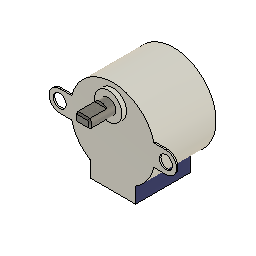
28BYJ-48 – 5V Stepper Motor (Autodesk Fusion 360 design; units mm, degrees)
Autodesk Fusion 360 part; units mm, degrees
sketch "Sketch1" plane through (0, 0, 0) normal (0, 1, 0) x (1, 0, 0)
  line L0 (-7.5, 17) -> (0, 17)
  line L1 (-7.5, 17) -> (-7.5, 11.8216)
  line L2 (-17.5, -3.5) -> (-13.5554, -3.5)
  circle A0 centre (-17.5, 0) radius 2.15
  line L3 (-17.5, 3.5) -> (-13.5554, 3.5)
  arc A1 (-7.5, 11.8216) -> (0, -14) centre (0, 0) ccw
  arc A2 (-17.5, 3.5) -> (-17.5, -3.5) centre (-17.5, 0) ccw
  arc A3 (0, -3.5) -> (0, -12.5) centre (0, -8) ccw
  arc A4 (0, 13.6015) -> (0, -13.6015) centre (0, 0) ccw
  arc A5 (0, -5.5) -> (0, -10.5) centre (0, -8) ccw
  line L4 (0, -9.5) -> (-2, -9.5)
  line L5 (-2, -6.5) -> (0, -6.5)
  line L6 (17.5, 3.5) -> (13.5554, 3.5)
  arc A6 (0, -14) -> (7.5, 11.8216) centre (0, 0) ccw
  arc A7 (17.5, -3.5) -> (17.5, 3.5) centre (17.5, 0) ccw
  arc A8 (0, -10.5) -> (0, -5.5) centre (0, -8) ccw
  line L7 (7.5, 17) -> (0, 17)
  line L8 (7.5, 17) -> (7.5, 11.8216)
  line L9 (2, -6.5) -> (0, -6.5)
  line L10 (0, -9.5) -> (2, -9.5)
  line L11 (17.5, -3.5) -> (13.5554, -3.5)
  arc A9 (0, -13.6015) -> (0, 13.6015) centre (0, 0) ccw
  arc A10 (0, -12.5) -> (0, -3.5) centre (0, -8) ccw
  circle A11 centre (17.5, 0) radius 2.15
  circle A12 centre (0, 0) radius 14
  dimension "d1" = 28
  dimension "d2" = 17
  dimension "d3" = 7.5
  dimension "d4" = 3.5
  dimension "d5" = 4.3
  dimension "d6" = 17.5
  dimension "d7" = 7
  dimension "d8" = 9
  dimension "d9" = 8
  dimension "d10" = 5
  measures "d1" diameter of A1
  measures "d2" distance of A1.centre L0
  measures "d3" distance of A1.centre L1
  measures "d4" distance of A1.centre L2
  measures "d5" diameter of A0
  measures "d6" distance of A1.centre
  measures "d7" diameter of A2
  measures "d8" diameter of A3
  measures "d9" distance of A1.centre
  measures "d10" diameter of A5
extrude "Extrude4" add sketch "Sketch1" along normal blind 0.5 contours L0 L1 L7 L8 A12 | A1 A6 A12 | L2 L3 A1 A2 A12 | L6 A6 A7 L11 A12 | A4 A9 makes body 1
extrude "Extrude5" add sketch "Sketch1" along normal blind 20 contours A1 A6 A12 | A3 A10 | A4 A9 | A5 L5 A8 L9 | A5 L4 L5 A8 L9 L10 | A5 L4 A8 L10 bodies 1
extrude "Extrude6" add sketch "Sketch1" along normal blind 18 contours L0 L1 L7 L8 A12 bodies 1
extrude "Extrude7" add sketch "Sketch1" against normal blind 1.5 separate body contours A3 A10 makes body 2
extrude "Extrude8" add sketch "Sketch1" against normal blind 10 separate body contours A5 L4 L5 A8 L9 L10 makes body 3
extrude "Extrude9" add sketch "Sketch1" against normal blind 4 contours A5 L5 A8 L9 | A5 L4 A8 L10 bodies 1 2 3
chamfer "Chamfer2" distance 0.5 angle 45 4 edges at (0, -10, 9.5) (2.5, -10, 8) (0, -10, 6.5) (-2.5, -10, 8) on bodies 1 3
sketch "Sketch2" plane through (0, 20, 0) normal (0, 1, 0) x (-1, 0, 0)
  circle A0 centre (0, 0) radius 14
  line L0 (0, 0) -> (-7.5555, 0)
  line L1 (-7.5555, 0) -> (7.5587, 0) construction
  line L2 (7.5587, 0) -> (7.5587, 3.5) construction
  line L3 (7.5587, 3.5) -> (-7.5555, 3.5) construction
  line L4 (-7.5555, 3.5) -> (-7.5555, 0) construction
  circle A1 centre (0, 0) radius 14
  text T0 "28BYJ-48" font "Arial" height 3.5 align ink ink in box 0 x 0 at (-7.5455, 0.02) x (1, 0) y (0, 1) spacing 1 height is em
extrude "Extrude10" cut sketch "Sketch2" against normal blind 0.5 text T0 bodies 1
equation "d6 = ( 35 / 2 ) * 1 mm"
named bodies: "Motor Body"
